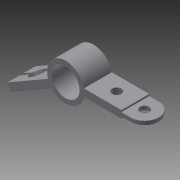
# Autodesk Inventor part: HW 8 Part 4
Saved by Autodesk Inventor 2015 (Build 190159000, 159)
## iProperties
Created: 2016-03-08
Part Number: HW 8 Part 4
Material: Generic
Document SubType Name: Modeling
Designer: Melissa
Density: 1 g/cm^3
Appearance: Default
Author: Melissa
Autodesk Inventor part; units mm, degrees
ref_plane "YZ Plane" through (0, 0, 0) normal (1, 0, 0) x (0, 1, 0)
ref_plane "XZ Plane" through (0, 0, 0) normal (0, 1, 0) x (-1, 0, 0)
ref_plane "XY Plane" through (0, 0, 0) normal (0, 0, 1) x (1, 0, 0)
sketch "Sketch1" plane through (0, 0, 0) normal (0, 0, 1) x (1, 0, 0)
  circle A0 centre (0, 0) radius 9.525
  line L0 (38.1, 1.27) -> (38.1, 2.54)
  line L1 (38.1, -1.27) -> (38.1, -2.54)
  line L2 (38.1, -2.54) -> (12.4434, -2.54)
  line L3 (38.1, 2.54) -> (12.4434, 2.54)
  line L4 (38.1, 0) -> (44.45, 0)
  line L5 (44.45, 0) -> (44.45, 1.27)
  line L6 (44.45, 1.27) -> (38.1, 1.27)
  line L7 (44.45, -1.27) -> (44.45, 0)
  line L8 (44.45, -1.27) -> (38.1, -1.27)
  line L9 (-38.4948, -22.225) -> (-37.2248, -24.4247)
  line L10 (-37.2248, -24.4247) -> (-9.5063, -8.4214)
  line L11 (-38.4948, -22.225) -> (-39.7648, -20.0253)
  line L12 (-39.7648, -20.0253) -> (-12.0463, -4.022)
  arc A1 (12.4434, 2.54) -> (-12.0463, -4.022) centre (0, 0) ccw
  arc A2 (-9.5063, -8.4214) -> (12.4434, -2.54) centre (0, 0) ccw
  dimension "d1" = 19.05
  dimension "d5" = 38.1
  dimension "d6" = 2.54
  dimension "d7" = 2.54
  dimension "d8" = 6.35
  dimension "d9" = 1.27
  dimension "d11" = 44.45
  dimension "d12" = 2.54
  dimension "d13" = 2.54
  dimension "d36" = 12.7
  constraints: 26 end point, 4 point on circle, 3 centre point, 3 perpendicular, 2 coincident, 2 parallel, 2 vertical, 1 point on line
  measures "d1" diameter of A0
  measures "d5" distance of A0.centre L4.start
  measures "d6" distance of L4.start L0.end
  measures "d7" distance of L4.start L1.end
  measures "d8" distance of L4.start L4.end
  measures "d9" distance of L4.end L5.end
  measures "d11" distance of A0.centre L9.start
  measures "d12" distance of L9.start L9.end
  measures "d13" distance of L9.start L11.end
  measures "d36" radius of A1
extrude "Extrusion1" add sketch "Sketch1" along normal mid plane 19.05
sketch "Sketch4" plane through (38.1, 1.27, 9.525) normal (0, 1, 0) x (1, 0, 0)
  arc A0 (6.35, 0) -> (6.35, 19.05) centre (6.35, 9.525) ccw
  line L0 (6.35, 19.05) -> (6.35, 0)
  line L1 (0, 0) -> (6.35, 0) projected
  point P0 (-38.1, 9.525)
  dimension "d16" = 9.525
  constraints: 2 end point, 2 point on circle, 1 centre point, 1 perpendicular
  measures "d16" radius of A0
extrude "Extrusion2" add sketch "Sketch4" against normal blind 2.54
sketch "Sketch5" plane through (38.1, 1.27, 9.525) normal (0, 1, 0) x (1, 0, 0)
  arc A0 (6.35, 0) -> (6.35, 19.05) centre (6.35, 9.525) ccw projected
  circle A1 centre (6.35, 9.525) radius 3.175
  circle A2 centre (-11.5739, 9.525) radius 3.175
  point P0 (-38.1, 9.525)
  dimension "d19" = 6.35
  constraints: 2 centre point, 1 coincident
  measures "d19" diameter of A1
extrude "Extrusion3" cut sketch "Sketch5" against normal through all contours A1
sketch "Sketch6" plane through (12.4434, 2.54, 9.525) normal (0, 1, 0) x (1, 0, 0)
  circle A0 centre (12.9566, 9.525) radius 3.175
  line L0 (25.6566, 19.05) -> (0, 19.05) projected
  line L1 (25.6566, 19.05) -> (25.6566, 0) projected
  point P0 (-12.4434, 9.525)
  dimension "d23" = 6.35
  dimension "d24" = 9.525
  dimension "d25" = 12.7
  constraints: 1 centre point
  measures "d23" diameter of A0
  measures "d24" distance from line of L0 A0.centre
  measures "d25" distance from line of L1 A0.centre
extrude "Extrusion4" cut sketch "Sketch6" against normal through all
sketch "Sketch7" plane through (-39.7648, -20.0253, 9.525) normal (-0.5, 0.866, 0) x (0.866, 0.5, 0)
  arc A0 (7.7813, 8.255) -> (7.7813, 10.795) centre (12.7, 9.525) ccw
  line L0 (0, 0) -> (0, 19.05) projected
  line L1 (0, 19.05) -> (32.0066, 19.05) projected
  line L2 (7.7813, 10.795) -> (0, 10.795)
  line L3 (7.7813, 8.255) -> (0, 8.255)
  line L4 (0, 10.795) -> (0, 8.255)
  point P0 (44.45, 9.525)
  dimension "d28" = 10.16
  dimension "d29" = 12.7
  dimension "d33" = 9.525
  constraints: 6 end point, 2 point on circle, 1 centre point, 1 vertical
  measures "d28" diameter of A0
  measures "d29" distance from line of L0 A0.centre
  measures "d33" distance from line of L1 A0.centre
extrude "Extrusion5" cut sketch "Sketch7" against normal through all
body "Solid1"
